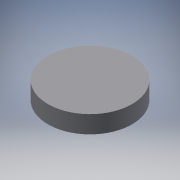
# Autodesk Inventor part: Heat-Sink
Saved by Autodesk Inventor 2017 (Build 210142000, 142)
## iProperties
Created: 2017-09-01
Part Number: Heat-Sink
Material: Generic
Document SubType Name: Modeling
Designer: tshum
Density: 1 g/cm^3
Appearance: Default
Author: tshum
Autodesk Inventor part; units mm, degrees
ref_plane "YZ Plane" through (0, 0, 0) normal (1, 0, 0) x (0, 1, 0)
ref_plane "XZ Plane" through (0, 0, 0) normal (0, 1, 0) x (-1, 0, 0)
sketch "Sketch1" plane through (0, 0, 0) normal (0, 1, 0) x (-1, 0, 0)
  circle A0 centre (0, 0) radius 76.2
  dimension "d0" = 152.4
  constraints: 1 centre point, 1 coincident
  measures "d0" diameter of A0
extrude "Extrusion1" add sketch "Sketch1" along normal blind 31.75
ref_plane "Work Plane1" through (0, 0, 76.2) normal (0, 0, 1) x (1, 0, 0)
sketch "Sketch2" plane through (0, 0, 76.2) normal (0, 0, 1) x (1, 0, 0)
  point P0 (0, 0)
  point P1 (0, 15.875)
  dimension "d4" = 15.875
  constraints: 1 vertical alignment
  measures "d4" distance of point (0, 0) point (0, 15.875)
hole "Hole1" at (0, 15.875, 76.2) direction (0, 0, -1) diameter 6.4008 depth 25.4 tip angle 118 thread size "5/16-18 UNC" class "2B" standard "ANSI Unified Screw Threads"
pattern_circular "Circular Pattern1" count 3 over 360 about axis through (0, 31.75, 0) along (0, 1, 0) of "Hole1"
body "Solid1"
